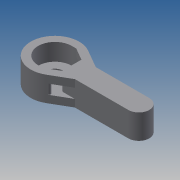
# Autodesk Inventor part: distal arm 2
Saved by Autodesk Inventor 2013 (Build 170138000, 138)
## iProperties
Created: 2017-04-05
Part Number: distal arm 2
Material: Generic
Document SubType Name: Modeling
Designer: employee
Density: 1 g/cm^3
Author: employee
Autodesk Inventor part; units mm, degrees
ref_plane "YZ Plane" through (0, 0, 0) normal (1, 0, 0) x (0, 1, 0)
ref_plane "XZ Plane" through (0, 0, 0) normal (0, 1, 0) x (-1, 0, 0)
ref_plane "XY Plane" through (0, 0, 0) normal (0, 0, 1) x (1, 0, 0)
sketch "Sketch1" plane through (0, 0, 0) normal (0, 0, 1) x (1, 0, 0)
  line L0 (0, 14) -> (112.5, 14)
  arc A0 (112.5, -14) -> (112.5, 14) centre (112.5, 0) ccw
  line L1 (112.5, -14) -> (0, -14)
  arc A1 (0, 14) -> (0, -14) centre (0, 0) ccw
  dimension "d0" = 28
  dimension "d2" = 112.5
  constraints: 4 end point, 4 point on circle, 4 tangent, 2 centre point, 1 coincident, 1 horizontal, 1 parallel
  measures "d0" distance between parallel lines of L1 L0
  measures "d2" distance of L1.start L1.end
extrude "Extrusion1" add sketch "Sketch1" along normal blind 33
sketch "Sketch2" plane through (0, 0, 33) normal (0, 0, 1) x (1, 0, 0)
  arc A0 (0, 14) -> (0, -14) centre (0, 0) ccw projected
  circle A1 centre (0, 0) radius 32.5
  dimension "d5" = 65
  constraints: 1 centre point, 1 coincident
  measures "d5" diameter of A1
extrude "Extrusion2" add sketch "Sketch2" against normal up to surface (33 mm away)
sketch "Sketch3" plane through (0, 0, 33) normal (0, 0, 1) x (1, 0, 0)
  arc A0 (29.33, 14) -> (29.33, -14) centre (0, 0) ccw projected
  circle A1 centre (0, 0) radius 22.5
  dimension "d10" = 45
  constraints: 1 centre point, 1 coincident
  measures "d10" diameter of A1
extrude "Extrusion3" cut sketch "Sketch3" against normal blind 23
sketch "Sketch4" plane through (0, 0, 33) normal (0, 0, 1) x (1, 0, 0)
  line L0 (29.33, -14) -> (112.5, -14) projected
  line L1 (112.5, 14) -> (29.33, 14) projected
  arc A0 (29.33, 14) -> (29.33, -14) centre (0, 0) ccw projected
  line L2 (16.25, 28.1458) -> (40.7513, 14)
  line L3 (16.25, -28.1458) -> (40.7513, -14)
  circle A1 centre (0, 0) radius 22.5 projected
  line L4 (11.25, -19.4856) -> (27.6862, -9.9961)
  dimension "d16" = 60
  constraints: 6 end point, 2 point on circle, 2 point on line, 2 tangent, 1 parallel, 1 vertical alignment, 3 other
  measures "d16" angle of L3 L2
extrude "Extrusion4" add sketch "Sketch4" against normal up to surface (33 mm away) contours L0 L3 A0 | L1 A0 L2
sketch "Sketch5" plane through (0, 0, 10) normal (0, 0, 1) x (1, 0, 0)
  circle A0 centre (0, 0) radius 22.5 projected
  circle A1 centre (0, 0) radius 22.5 projected
  line L0 (40.7513, -14) -> (112.5, -14) projected
  arc A2 (112.5, -14) -> (112.5, 14) centre (112.5, 0) ccw projected
  line L1 (112.5, 14) -> (40.7513, 14) projected
  line L2 (40.7513, 14) -> (16.25, 28.1458) projected
  arc A3 (16.25, 28.1458) -> (16.25, -28.1458) centre (0, 0) ccw projected
  line L3 (16.25, -28.1458) -> (40.7513, -14) projected
  line L4 (0, -22.5) -> (40.7513, -22.5)
  line L5 (40.7513, -22.5) -> (40.7513, -14)
  line L6 (40.7513, -14) -> (0, -14)
  line L7 (0, -14) -> (0, -22.5)
  constraints: 8 end point, 2 horizontal, 2 parallel, 2 vertical alignment, 1 perpendicular, 2 other
extrude "Extrusion5" cut sketch "Sketch5" along normal blind 13 contours L7 L6 A0 | A0 L6 L3 L4 | L3 L5 L4 picked at (10.5546, -15.1914)
sketch "Sketch6" plane through (0, 0, 33) normal (0, 0, 1) x (1, 0, 0)
  circle A0 centre (0, 0) radius 22.5 projected
  line L0 (112.5, 14) -> (40.7513, 14) projected
  arc A1 (16.25, 28.1458) -> (16.25, -28.1458) centre (0, 0) ccw projected
  line L1 (16.25, -28.1458) -> (40.7513, -14) projected
  line L2 (0, -22.5) -> (6.0289, -22.5)
  line L3 (6.0289, -22.5) -> (22.5, -12.9904)
  line L4 (22.5, -12.9904) -> (22.5, 0)
  line L5 (22.5, 0) -> (0, 0)
  line L6 (0, 0) -> (0, -22.5)
  dimension "d19" = 10
  constraints: 10 end point, 3 parallel, 2 vertical, 1 perpendicular, 1 vertical alignment, 1 other
  measures "d19" distance between parallel lines of L3 L1
extrude "Extrusion6" cut sketch "Sketch6" against normal up to surface (23 mm away) contours L4 L3 A0 | A0 L6 L5 | A0 L3 L2 picked at (8.7685, -12.0688)
sketch "Sketch7" plane through (0, 0, 10) normal (0, 0, 1) x (1, 0, 0)
  line L0 (40.7513, -14) -> (20.7513, -14) projected
  line L1 (22.5, -12.9904) -> (20.7513, -14) projected
  line L2 (22.5, -12.9904) -> (22.5, -14)
  constraints: 2 end point, 1 perpendicular, 1 point on line
extrude "Extrusion7" cut sketch "Sketch7" along normal up to surface (13 mm away)
mirror "Mirror1" about plane through (0, 0, 0) normal (0, 1, 0) of "Extrusion7", "Extrusion6", "Extrusion5"
fillet "Fillet1" radius 2.5 4 edges at (22.5, -14, 16.5) (22.5, 14, 16.5) (26.0289, -22.5, 16.5) (26.0289, 22.5, 16.5)
sketch "Sketch8" plane through (0, 0, 10) normal (0, 0, 1) x (1, 0, 0)
  arc A0 (0, 22.5) -> (0, -22.5) centre (0, 0) ccw projected
  circle A1 centre (0, 0) radius 11
  dimension "d25" = 22
  constraints: 1 centre point, 1 coincident
  measures "d25" diameter of A1
extrude "Extrusion8" cut sketch "Sketch8" against normal blind 7
sketch "Sketch9" plane through (0, 0, 3) normal (0, 0, 1) x (1, 0, 0)
  circle A0 centre (0, 0) radius 11 projected
  circle A1 centre (0, 0) radius 7.5
  dimension "d29" = 15
  constraints: 1 centre point, 1 coincident
  measures "d29" diameter of A1
extrude "Extrusion9" cut sketch "Sketch9" against normal through all contours A1
fillet "Fillet2" radius 3.5 1 edges at (-7.5, 0, 3)
sketch "Sketch10" plane through (0, 0, 0) normal (0, 0, -1) x (-1, 0, 0)
  arc A0 (-112.5, 14) -> (-112.5, -14) centre (-112.5, 0) ccw projected
  circle A1 centre (-112.5, 0) radius 6
  circle A2 centre (-72.5, 0) radius 6
  dimension "d34" = 40
  dimension "d35" = 12
  constraints: 2 centre point, 1 coincident, 1 equal radius, 1 horizontal alignment
  measures "d34" distance of A0.centre A2.centre
  measures "d35" diameter of A2
extrude "Extrusion10" cut sketch "Sketch10" against normal through all
sketch "Sketch11" plane through (0, 0, 0) normal (0, 0, -1) x (-1, 0, 0)
  circle A0 centre (-112.5, 0) radius 6 projected
  circle A1 centre (-72.5, 0) radius 6 projected
  arc A2 (-16.25, -28.1458) -> (-16.25, 28.1458) centre (0, 0) ccw projected
  line L0 (-40.7513, 14) -> (-112.5, 14) projected
  arc A3 (-112.5, 14) -> (-112.5, -14) centre (-112.5, 0) ccw projected
  line L1 (-112.5, -14) -> (-40.7513, -14) projected
  line L2 (-60, -14) -> (-60, -6)
  line L3 (-60, -6) -> (-30, -6)
  line L4 (-30, -6) -> (-30, 6)
  line L5 (-30, 6) -> (-60, 6)
  line L6 (-60, 6) -> (-60, 14)
  point P0 (-45, -6)
  dimension "d38" = 8
  dimension "d39" = 30
  dimension "d40" = 45
  constraints: 10 end point, 3 perpendicular, 2 equal length, 2 parallel, 2 point on line, 1 coincident, 1 midpoint
  measures "d38" distance between parallel lines of L3 L1
  measures "d39" distance of L4.end L5.end
  measures "d40" horizontal distance of point (0, 0) point (-45, -6)
extrude "Extrusion11" cut sketch "Sketch11" against normal through all
sketch "Sketch12" plane through (40.7513, 14, 10) normal (0, 1, 0) x (1, 0, 0)
  line L0 (19.2487, -23) -> (19.2487, 10) projected
  line L1 (19.2487, -23) -> (0, -23) projected
  line L2 (7.2487, -18.5) -> (7.2487, -10.5)
  line L3 (7.2487, -10.5) -> (7.2487, -2.5)
  line L4 (7.2487, -2.5) -> (7.2487, 5.5)
  circle A0 centre (7.2487, 5.5) radius 1.75
  circle A1 centre (7.2487, -2.5) radius 1.75
  circle A2 centre (7.2487, -10.5) radius 1.75
  circle A3 centre (7.2487, -18.5) radius 1.75
  line L5 (14.2487, -14.5) -> (14.2487, -6.5)
  line L6 (14.2487, -6.5) -> (14.2487, 1.5)
  circle A4 centre (14.2487, -6.5) radius 1.75
  circle A5 centre (14.2487, 1.5) radius 1.75
  circle A6 centre (14.2487, -14.5) radius 1.75
  circle A7 centre (-2.7513, -6.5) radius 1.75
  line L7 (-10.7513, 10) -> (-10.7513, -23) projected
  line L8 (0, 10) -> (19.2487, 10) projected
  line L9 (0, 10) -> (0, 0) projected
  line L10 (0, 0) -> (-15.7513, 0) projected
  line L11 (-15.7513, -13) -> (-15.7513, 0) projected
  line L12 (0, -13) -> (-15.7513, -13) projected
  line L13 (0, -13) -> (0, -23) projected
  point P0 (-40.7513, 10)
  point P1 (7.2487, -6.5)
  point P2 (19.2487, -6.5)
  point P3 (-10.7513, -6.5)
  dimension "d43" = 8
  dimension "d45" = 3.5
  dimension "d47" = 5
  dimension "d48" = 7
  dimension "d59" = 8
  constraints: 10 end point, 8 centre point, 7 coincident, 7 equal radius, 4 equal length, 4 parallel, 3 horizontal alignment, 3 midpoint, 1 perpendicular
  measures "d43" distance of L2.end L3.end
  measures "d45" diameter of A3
  measures "d47" distance between parallel lines of L5 L0
  measures "d48" distance between parallel lines of L5 L3
  measures "d59" distance from line of A7.centre L7
extrude "Extrusion12" cut sketch "Sketch12" against normal through all contours A2 L3 L2 | L2 L3 A2 | A1 L4 L3 | L3 L4 A1 | A0 | A3 | A4 L6 L5 | L5 L6 A4 | A5 | A6 | A7
sketch "Sketch13" plane through (40.7513, 14, 10) normal (0, 1, 0) x (1, 0, 0)
  circle A0 centre (14.2487, 1.5) radius 1.75 projected
  circle A1 centre (7.2487, -18.5) radius 1.75 projected
  circle A2 centre (7.2487, -2.5) radius 1.75 projected
  circle A3 centre (7.2487, 5.5) radius 1.75 projected
  circle A4 centre (7.2487, -10.5) radius 1.75 projected
  circle A5 centre (14.2487, -6.5) radius 1.75 projected
  circle A6 centre (14.2487, -14.5) radius 1.75 projected
  circle A7 centre (7.2487, 5.5) radius 3
  circle A8 centre (14.2487, 1.5) radius 3
  circle A9 centre (7.2487, -2.5) radius 3
  circle A10 centre (14.2487, -6.5) radius 3
  circle A11 centre (14.2487, -14.5) radius 3
  circle A12 centre (7.2487, -10.5) radius 3
  circle A13 centre (7.2487, -18.5) radius 3
  circle A14 centre (-2.7513, -6.5) radius 1.75 projected
  circle A15 centre (-2.7513, -6.5) radius 3
  point P0 (-40.7513, 10)
  dimension "d51" = 6
  constraints: 8 centre point, 7 equal radius, 1 coincident
  measures "d51" diameter of A7
extrude "Extrusion13" cut sketch "Sketch13" against normal blind 3
sketch "Sketch14" plane through (40.7513, -14, 0) normal (0, -1, 0) x (1, 0, 0)
  circle A0 centre (14.2487, 8.5) radius 1.75 projected
  circle A1 centre (7.2487, 28.5) radius 1.75 projected
  circle A2 centre (7.2487, 12.5) radius 1.75 projected
  circle A3 centre (7.2487, 4.5) radius 1.75 projected
  circle A4 centre (7.2487, 20.5) radius 1.75 projected
  circle A5 centre (14.2487, 16.5) radius 1.75 projected
  circle A6 centre (14.2487, 24.5) radius 1.75 projected
  line L0 (4.0733, 4.5) -> (5.661, 7.25)
  line L1 (5.661, 7.25) -> (8.8364, 7.25)
  line L2 (8.8364, 7.25) -> (10.4241, 4.5)
  line L3 (10.4241, 4.5) -> (8.8364, 1.75)
  line L4 (8.8364, 1.75) -> (5.661, 1.75)
  line L5 (5.661, 1.75) -> (4.0733, 4.5)
  line L6 (4.0733, 12.5) -> (5.661, 15.25)
  line L7 (5.661, 15.25) -> (8.8364, 15.25)
  line L8 (8.8364, 15.25) -> (10.4241, 12.5)
  line L9 (10.4241, 12.5) -> (8.8364, 9.75)
  line L10 (8.8364, 9.75) -> (5.661, 9.75)
  line L11 (5.661, 9.75) -> (4.0733, 12.5)
  line L12 (11.0733, 8.5) -> (12.661, 11.25)
  line L13 (12.661, 11.25) -> (15.8364, 11.25)
  line L14 (15.8364, 11.25) -> (17.4241, 8.5)
  line L15 (17.4241, 8.5) -> (15.8364, 5.75)
  line L16 (15.8364, 5.75) -> (12.661, 5.75)
  line L17 (12.661, 5.75) -> (11.0733, 8.5)
  line L18 (11.0733, 16.5) -> (12.661, 19.25)
  line L19 (12.661, 19.25) -> (15.8364, 19.25)
  line L20 (15.8364, 19.25) -> (17.4241, 16.5)
  line L21 (17.4241, 16.5) -> (15.8364, 13.75)
  line L22 (15.8364, 13.75) -> (12.661, 13.75)
  line L23 (12.661, 13.75) -> (11.0733, 16.5)
  line L24 (4.0733, 20.5) -> (5.661, 23.25)
  line L25 (5.661, 23.25) -> (8.8364, 23.25)
  line L26 (8.8364, 23.25) -> (10.4241, 20.5)
  line L27 (10.4241, 20.5) -> (8.8364, 17.75)
  line L28 (8.8364, 17.75) -> (5.661, 17.75)
  line L29 (5.661, 17.75) -> (4.0733, 20.5)
  line L30 (11.0733, 24.5) -> (12.661, 27.25)
  line L31 (12.661, 27.25) -> (15.8364, 27.25)
  line L32 (15.8364, 27.25) -> (17.4241, 24.5)
  line L33 (17.4241, 24.5) -> (15.8364, 21.75)
  line L34 (15.8364, 21.75) -> (12.661, 21.75)
  line L35 (12.661, 21.75) -> (11.0733, 24.5)
  line L36 (4.0733, 28.5) -> (5.661, 31.25)
  line L37 (5.661, 31.25) -> (8.8364, 31.25)
  line L38 (8.8364, 31.25) -> (10.4241, 28.5)
  line L39 (10.4241, 28.5) -> (8.8364, 25.75)
  line L40 (8.8364, 25.75) -> (5.661, 25.75)
  line L41 (5.661, 25.75) -> (4.0733, 28.5)
  circle A7 centre (-2.7513, 16.5) radius 1.75 projected
  line L42 (0.4241, 16.5) -> (-1.1636, 13.75)
  line L43 (-1.1636, 13.75) -> (-4.339, 13.75)
  line L44 (-4.339, 13.75) -> (-5.9267, 16.5)
  line L45 (-5.9267, 16.5) -> (-4.339, 19.25)
  line L46 (-4.339, 19.25) -> (-1.1636, 19.25)
  line L47 (-1.1636, 19.25) -> (0.4241, 16.5)
  point P0 (-40.7513, 0)
  dimension "d55" = 5.5
  constraints: 96 end point, 8 coincident, 8 horizontal, 7 parallel, 104 other
  measures "d55" distance between parallel lines of L28 L25
extrude "Extrusion14" cut sketch "Sketch14" against normal blind 4
body "Solid1"
